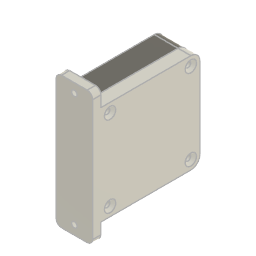
M5Stack UI Holder v3 (Autodesk Fusion 360 design; units mm, degrees)
Autodesk Fusion 360 part; units mm, degrees
note: some values were not read from the file. Set by a fixed rule: which sketch regions a step uses.
sketch "Sketch1" plane through (0, 0, 0) normal (0, 1, 0) x (1, 0, 0) in component "UI Holder"
  circle A0 centre (0, 0) radius 1.5
  circle A1 centre (0, -62) radius 1.5
  line L0 (0, 0) -> (0, -62) construction
  line L1 (-10, -67) -> (10, -67)
  line L2 (10, -67) -> (10, 5)
  line L3 (10, 5) -> (-10, 5)
  line L4 (-10, 5) -> (-10, -67)
  line L5 (0, 5) -> (0, 0) construction
  line L6 (0, -31) -> (10, -31) construction
  dimension "d1" = 3
  dimension "d2" = 3
  dimension "d3" = 62
  dimension "d4" = 72
  dimension "d5" = 20
  constraint coincident A0.centre L0.start
  constraint coincident A1.centre L0.end
  constraint vertical L0
  constraint horizontal L1
  constraint vertical L2
  constraint horizontal L3
  constraint vertical L4
  constraint midpoint L3 L5.start
  constraint vertical L5
  constraint midpoint L0 L6.start
  constraint midpoint L2 L6.end
  constraint horizontal L6
  measures "d1" diameter of A0
  measures "d2" diameter of A1
  measures "d3" vertical distance of A0.centre A1.centre
  measures "d4" distance of L1.end L2.end
  measures "d5" distance of L1.start L1.end
extrude "Extrude1" add sketch "Sketch1" along normal blind 4.5 makes body 1 in component "UI Holder"
fillet "Fillet1" radius 3 4 edges at (10, 2.25, 67) (10, 2.25, -5) (-10, 2.25, -5) (-10, 2.25, 67) on bodies 1 in component "UI Holder"
ref_plane "WorkPlane2" through (-10, 2.25, 31) normal (-1, 0, 0) x (0, 0, 1) in component "M5Stack Core"
sketch "Sketch3" plane through (-10, 2.25, 29) normal (-1, 0, 0) x (0, 1, 0) in component "M5Stack Core"
  line L0 (2.25, -35) -> (2.25, 31)
  line L1 (2.25, -29) -> (56.25, -29)
  line L2 (56.25, -29) -> (56.25, 25)
  line L3 (56.25, 25) -> (2.25, 25)
  line L4 (2.25, 25) -> (2.25, -29)
  line L5 (7.25, -24) -> (51.25, -24)
  line L6 (51.25, -24) -> (51.25, 20)
  line L7 (51.25, 20) -> (7.25, 20)
  line L8 (7.25, 20) -> (7.25, -24)
  line L9 (29.25, -29) -> (29.25, -24) construction
  line L10 (2.25, -2) -> (7.25, -2)
  circle A0 centre (7.25, -24) radius 1.5
  circle A1 centre (51.25, -24) radius 1.5
  circle A2 centre (7.25, 20) radius 1.5
  circle A3 centre (51.25, 20) radius 1.5
  point P0 (2.25, -2)
  point P1 (2.25, -2)
  dimension "d12" = 54
  dimension "d13" = 54
  dimension "d14" = 44
  dimension "d15" = 44
  dimension "d16" = 3
  dimension "d17" = 3
  dimension "d18" = 3
  dimension "d19" = 3
  constraint horizontal L1
  constraint vertical L2
  constraint horizontal L3
  constraint vertical L4
  constraint midpoint L4 P1
  constraint midpoint L0 P1
  constraint coincident P1 P0
  constraint horizontal L5
  constraint vertical L6
  constraint horizontal L7
  constraint vertical L8
  constraint midpoint L1 L9.start
  constraint midpoint L5 L9.end
  constraint midpoint L8 L10.end
  constraint horizontal L10
  constraint vertical L9
  constraint coincident L5.start L8.end
  constraint coincident L5.end L6.start
  constraint coincident L7.end L8.start
  constraint coincident L6.end L7.start
  measures "d12" distance of L1.start L1.end
  measures "d13" distance of L1.start L3.end
  measures "d14" distance of L5.start L5.end
  measures "d15" distance of L5.start L7.end
  measures "d16" diameter of A0
  measures "d17" diameter of A1
  measures "d18" diameter of A2
  measures "d19" diameter of A3
extrude "Extrude1'" add sketch "Sketch3" against normal blind 2 separate body contours L0 L1 L2 L3 L4 | L5 L8 A0 | L5 L8 A0 | L5 L6 L7 L8 A0 A1 A2 A3 | L5 L6 A1 | L5 L6 A1 | L7 L8 A2 | L7 L8 A2 | L6 L7 A3 | L6 L7 A3 makes body 2 in component "M5Stack Core"
fillet "Fillet1'" radius 5 4 edges at (-9, 58.5, 58) (-9, 4.5, 58) (-9, 4.5, 4) (-9, 58.5, 4) on bodies 2 in component "M5Stack Core"
extrude "Extrude2" add sketch "Sketch3" against normal blind 11 from surface at -2 bodies 2 in component "M5Stack Core"
fillet "Fillet2" radius 5 4 edges at (-2.5, 58.5, 58) (-2.5, 4.5, 58) (-2.5, 4.5, 4) (-2.5, 58.5, 4) on bodies 2 in component "M5Stack Core"
ref_plane "WorkPlane1" through (3, 31.5, 31) normal (1, 0, 0) x (0, 0, -1) in component "M5Stack UI PCB"
sketch "Sketch1 (2)" plane through (3, 31.5, 29) normal (1, 0, 0) x (0, 1, 0) in component "M5Stack UI PCB"
  circle A0 centre (22, 24) radius 1.5
  circle A1 centre (-22, 24) radius 1.5
  circle A2 centre (-22, -20) radius 1.5
  circle A3 centre (22, -20) radius 1.5
  line L0 (-24, 27) -> (24, 27)
  line L1 (25, 26) -> (25, -22)
  line L2 (24, -23) -> (-24, -23)
  line L3 (-25, -22) -> (-25, 26)
  line L4 (-22, 24) -> (-22, -20) construction
  line L5 (-22, -20) -> (22, -20) construction
  line L6 (-22, 2) -> (-25, 2) construction
  line L7 (0, -20) -> (0, -23) construction
  line L8 (-24, 27) -> (-25, 26)
  line L9 (-24, -23) -> (-25, -22)
  line L10 (24, -23) -> (25, -22)
  line L11 (25, 26) -> (24, 27)
  line L12 (-2.6, -15.4) -> (14.4, -15.4)
  line L13 (14.4, -15.4) -> (14.4, -23)
  line L14 (14.4, -23) -> (-2.6, -23)
  line L15 (-2.6, -23) -> (-2.6, -15.4)
  line L16 (-16.2, -15.4) -> (-4.2, -15.4)
  line L17 (-4.2, -15.4) -> (-4.2, -23)
  line L18 (-4.2, -23) -> (-16.2, -23)
  line L19 (-16.2, -23) -> (-16.2, -15.4)
  line L20 (-16.2, -19.2) -> (-25, -19.2) construction
  line L21 (14.4, -19.2) -> (25, -19.2) construction
  point P0 (-25, 27)
  point P1 (25, 27)
  point P2 (25, -23)
  point P3 (-25, -23)
  point P4 (0, -23)
  point P5 (-25, 2)
  dimension "d30" = 50
  dimension "d31" = 50
  dimension "d32" = 1
  dimension "d33" = 1
  dimension "d34" = 1
  dimension "d35" = 1
  dimension "d36" = 1
  dimension "d37" = 1
  dimension "d38" = 1
  dimension "d39" = 1
  dimension "d42" = 17
  dimension "d43" = 7.6
  dimension "d44" = 12
  dimension "d45" = 7.6
  dimension "d46" = 8.8
  dimension "d47" = 10.6
  constraint horizontal L0
  constraint vertical L1
  constraint horizontal L2
  constraint vertical L3
  constraint coincident A1.centre L4.start
  constraint coincident A2.centre L4.end
  constraint coincident A3.centre L5.end
  constraint midpoint L4 L6.start
  constraint midpoint L5 L7.start
  constraint vertical L7
  constraint horizontal L6
  constraint coincident L3 P5
  constraint coincident P0 L0
  constraint coincident P0 L3
  constraint coincident L2 P4
  constraint coincident P3 L2
  constraint coincident P3 L3
  constraint coincident P2 L2
  constraint coincident P2 L1
  constraint coincident P1 L1
  constraint coincident P1 L0
  constraint midpoint L2 P4
  constraint coincident P4 L7.end
  constraint midpoint L3 P5
  constraint coincident P5 L6.end
  constraint horizontal L12
  constraint vertical L13
  constraint horizontal L14
  constraint vertical L15
  constraint horizontal L16
  constraint vertical L17
  constraint horizontal L18
  constraint vertical L19
  constraint collinear L2 L18
  constraint collinear L2 L14
  constraint midpoint L19 L20.start
  constraint perpendicular L19 L20
  constraint coincident L3 L20.end
  constraint midpoint L13 L21.start
  constraint coincident L1 L21.end
  constraint perpendicular L1 L21
  measures "d30" distance of P0 P1
  measures "d31" distance of P0 P3
  measures "d32" distance of P0 L0.start
  measures "d33" distance of P0 L3.end
  measures "d34" distance of P3 L2.end
  measures "d35" distance of P3 L3.start
  measures "d36" distance of P2 L2.start
  measures "d37" distance of P2 L1.end
  measures "d38" distance of P1 L1.start
  measures "d39" distance of P1 L0.end
  measures "d42" distance of L12.start L12.end
  measures "d43" distance of L12.start L14.end
  measures "d44" distance of L16.start L16.end
  measures "d45" distance of L16.start L18.end
  measures "d46" distance of L20.start L20.end
  measures "d47" distance of L21.start L21.end
extrude "Extrude1''" add sketch "Sketch1 (2)" against normal blind 1.6 separate body makes body 3 in component "M5Stack UI PCB"
extrude "Extrude2'" add sketch "Sketch1 (2)" along normal blind 5 contours L2 L16 L17 L18 L19 | L2 L12 L13 L14 L15 bodies 3 in component "M5Stack UI PCB"
ref_plane "WorkPlane1" through (3, 31.5, 31) normal (1, 0, 0) x (0, 0, -1) in component "UI Holder"
sketch "Sketch2" plane through (3, 31.5, 29) normal (1, 0, 0) x (0, 1, 0) in component "UI Holder"
  circle A0 centre (-22, 24) radius 1.5
  circle A1 centre (22, 24) radius 1.5
  circle A2 centre (22, -20) radius 1.5
  circle A3 centre (-22, -20) radius 1.5
  arc A4 (27, 24) -> (22, 29) centre (22, 24) ccw
  arc A5 (-22, 29) -> (-27, 24) centre (-22, 24) ccw
  line L0 (-27, 29) -> (27, 29)
  line L1 (-27, -25) -> (-27, 29)
  line L2 (27, 29) -> (27, -25)
  line L3 (27, -25) -> (-27, -25)
  arc A6 (22, -25) -> (27, -20) centre (22, -20) ccw
  arc A7 (-27, -20) -> (-22, -25) centre (-22, -20) ccw
  line L4 (-22, 29) -> (22, 29)
  line L5 (27, 24) -> (27, -20)
  line L6 (22, -25) -> (-22, -25)
  line L7 (-27, -20) -> (-27, 24)
  arc A8 (-22, 28) -> (-26, 24) centre (-22, 24) ccw
  line L8 (-26, -20) -> (-26, 24)
  arc A9 (-26, -20) -> (-22, -24) centre (-22, -20) ccw
  line L9 (22, -24) -> (-22, -24)
  arc A10 (22, -24) -> (26, -20) centre (22, -20) ccw
  line L10 (26, 24) -> (26, -20)
  arc A11 (26, 24) -> (22, 28) centre (22, 24) ccw
  line L11 (-22, 28) -> (22, 28)
  circle A12 centre (-22, 24) radius 3
  line L12 (-22, 28) -> (-22, 27)
  line L13 (-26, 24) -> (-25, 24)
  circle A13 centre (22, 24) radius 3
  line L14 (22, 28) -> (22, 27)
  line L15 (26, 24) -> (25, 24)
  circle A14 centre (22, -20) radius 3
  circle A15 centre (-22, -20) radius 3
  line L16 (22, -24) -> (22, -23)
  line L17 (26, -20) -> (25, -20)
  line L18 (-22, -24) -> (-22, -23)
  line L19 (-26, -20) -> (-25, -20)
  arc A16 (-22, 29.5) -> (-27.5, 24) centre (-22, 24) ccw
  line L20 (-27.5, -20) -> (-27.5, 24)
  arc A17 (-27.5, -20) -> (-22, -25.5) centre (-22, -20) ccw
  line L21 (22, -25.5) -> (-22, -25.5)
  arc A18 (22, -25.5) -> (27.5, -20) centre (22, -20) ccw
  line L22 (27.5, 24) -> (27.5, -20)
  arc A19 (27.5, 24) -> (22, 29.5) centre (22, 24) ccw
  line L23 (-22, 29.5) -> (22, 29.5)
  dimension "d51" = 1
  dimension "d55" = 1.5
  dimension "d56" = 1.5
  dimension "d57" = 1.5
  dimension "d58" = 1.5
  dimension "d76" = -0.5
  constraint coincident A5.start L4.start
  constraint coincident A4.end L4.end
  constraint coincident A4.start L5.start
  constraint coincident A6.end L5.end
  constraint coincident A6.start L6.start
  constraint coincident A7.end L6.end
  constraint coincident A7.start L7.start
  constraint coincident A5.end L7.end
  constraint coincident A12 L12.end
  constraint perpendicular L11 L12
  constraint coincident A12 L13.end
  constraint perpendicular L8 L13
  constraint coincident A13 L14.end
  constraint perpendicular L11 L14
  constraint coincident A13 L15.end
  constraint perpendicular L10 L15
  constraint coincident A14 L16.end
  constraint perpendicular L9 L16
  constraint coincident A14 L17.end
  constraint perpendicular L10 L17
  constraint coincident A15 L18.end
  constraint perpendicular L9 L18
  constraint coincident A15 L19.end
  constraint perpendicular L8 L19
  measures "d55" distance of A0
  measures "d56" distance of A1
  measures "d57" distance of A2
  measures "d58" distance of A3
ref_plane "WorkPlane2" through (4.7, 31.5, 6) normal (0, 0, -1) x (0, -1, 0) in component "UI Holder"
sketch "Sketch3 (2)" plane through (3.7, 31.5, 6) normal (0, 0, -1) x (1, 0, 0) in component "UI Holder"
  line L0 (-0.7, 16.2) -> (4.3, 16.2)
  line L1 (4.3, 16.2) -> (4.3, 4.2)
  line L2 (-0.7, 4.2) -> (4.3, 4.2)
  line L3 (-0.7, 2.6) -> (4.3, 2.6)
  line L4 (4.3, 2.6) -> (4.3, -14.4)
  line L5 (-0.7, -14.4) -> (4.3, -14.4)
  line L6 (-0.7, 17) -> (5.1, 17)
  line L7 (5.1, 17) -> (5.1, 3.4)
  line L8 (-0.7, 3.4) -> (5.1, 3.4)
  line L9 (-0.7, 3.4) -> (5.1, 3.4)
  line L10 (5.1, 3.4) -> (5.1, -15.2)
  line L11 (-0.7, -15.2) -> (5.1, -15.2)
  line L12 (-0.7, 17) -> (-0.7, -15.2)
  dimension "d53" = -0.8
  dimension "d54" = -0.8
  constraint perpendicular L11 L12
extrude "Extrude2''" add sketch "Sketch2" along normal up to surface (7 mm away) contours A4 A5 L0 L1 L2 L3 A6 A7 L4 L5 L6 L7 | A5 L0 L1 A16 | L0 L1 A16 | L1 L3 A7 A17 | L1 L3 A17 bodies 1 in component "UI Holder"
extrude "Extrude3" add sketch "Sketch2" along normal up to surface (6.5 mm away) from surface at 0.5 contours A8 A12 L12 L13 | A11 A13 L14 L15 | A12 | A9 A15 L18 L19 | A13 | A15 | A10 A14 L16 L17 | A14 bodies 1 in component "UI Holder"
extrude "Extrude4" add sketch "Sketch2" against normal blind 2 from surface at 7 contours L8 L9 L10 L11 A12 L12 L13 A13 L14 L15 A14 A15 L16 L17 L18 L19 bodies 1 in component "UI Holder"
extrude "Extrude5" cut sketch "Sketch3 (2)" along normal blind 6 and the other way blind 4 bodies 1 in component "UI Holder"
chamfer "Chamfer1" distance 2 angle 45 2 edges at (-1.3985, 4.5, -0.5424) (-1.3985, 4.5, 61.4576) on bodies 1 in component "UI Holder"
extrude "Extrude6" cut sketch "Sketch2" against normal up to surface (13 mm away) contours A5 L0 L1 A16 | L1 L7 A16 L20 A17 | L1 L3 A7 A17 bodies 1 in component "UI Holder"
chamfer "Chamfer2" distance 1.6 angle 45 4 edges at (10, 8.1015, 52.4576) (10, 52.1015, 52.4576) (10, 52.1015, 8.4576) (10, 8.1015, 8.4576) on bodies 1 in component "UI Holder"
component "UI Holder" placed x (1, 0, 0) y (0, 1, 0) z (0, 0, 1) at (0, 0, 0)
component "M5Stack Core" placed x (1, 0, 0) y (0, 1, 0) z (0, 0, 1) at (0, 0, 0)
component "M5Stack UI PCB" placed x (1, 0, 0) y (0, 1, 0) z (0, 0, 1) at (0, 0, 0)
equation "d33 = d32"
equation "d35 = d34"
equation "d37 = d36"
equation "d39 = d38"
named bodies: "M5Stack UI Holder"
